Autodesk Fusion 360 part; units mm, degrees
note: some values were not read from the file. Set by a fixed rule: which face or edge a step refers to.
(part 2 of 3)
sketch "Sketch8" plane through (0, 0, 5) normal (0, 0, 1) x (-1, 0, 0)
  line L0 (-17, 136) -> (-35, 136)
  line L1 (-35, 136) -> (-35, 130)
  line L2 (-35, 130) -> (-17, 130)
  line L3 (-17, 130) -> (-17, 128)
  line L4 (-17, 128) -> (-35, 128)
  line L5 (-35, 128) -> (-35, 122)
  line L6 (-35, 122) -> (-17, 122)
  line L7 (-17, 122) -> (-17, 120)
  line L8 (-17, 120) -> (-35, 120)
  line L9 (-35, 120) -> (-35, 114)
  line L10 (-35, 114) -> (-17, 114)
  line L11 (-17, 114) -> (-17, 112)
  line L12 (-17, 112) -> (-35, 112)
  line L13 (-35, 112) -> (-35, 106)
  line L14 (-35, 106) -> (-17, 106)
  line L15 (-17, 106) -> (-17, 104)
  line L16 (-17, 104) -> (-35, 104)
  line L17 (-35, 104) -> (-35, 98)
  line L18 (-35, 98) -> (-17, 98)
  line L19 (-17, 98) -> (-17, 96)
  line L20 (-17, 96) -> (-35, 96)
  line L21 (-35, 96) -> (-35, 90)
  line L22 (-35, 90) -> (-17, 90)
  line L23 (-17, 90) -> (-17, 88)
  line L24 (-17, 88) -> (-35, 88)
  line L25 (-35, 88) -> (-35, 82)
  line L26 (-35, 82) -> (-17, 82)
  line L27 (-17, 82) -> (-17, 80)
  line L28 (-17, 80) -> (-35, 80)
  line L29 (-35, 80) -> (-35, 74)
  line L30 (-35, 74) -> (-17, 74)
  line L31 (-17, 74) -> (-17, 72)
  line L32 (-17, 72) -> (-35, 72)
  line L33 (-35, 72) -> (-35, 66)
  line L34 (-35, 66) -> (-17, 66)
  line L35 (-17, 66) -> (-17, 64)
  line L36 (-17, 64) -> (-35, 64)
  line L37 (-35, 64) -> (-35, 58)
  line L38 (-35, 58) -> (-17, 58)
  line L39 (-17, 58) -> (-17, 56)
  line L40 (-17, 56) -> (-35, 56)
  line L41 (-35, 56) -> (-35, 50)
  line L42 (-35, 50) -> (-17, 50)
  line L43 (-17, 50) -> (-17, 48)
  line L44 (-17, 48) -> (-35, 48)
  line L45 (-35, 48) -> (-35, 42)
  line L46 (-35, 42) -> (-17, 42)
  line L47 (-17, 42) -> (-17, 40)
  line L48 (-17, 40) -> (-35, 40)
  line L49 (-35, 40) -> (-35, 34)
  line L50 (-35, 34) -> (-17, 34)
  line L51 (-17, 34) -> (-17, 32)
  line L52 (-17, 32) -> (-35, 32)
  line L53 (-35, 32) -> (-35, 26)
  line L54 (-35, 26) -> (-17, 26)
  line L55 (-17, 26) -> (-17, 24)
  line L56 (-17, 24) -> (-35, 24)
  line L57 (-35, 24) -> (-35, 18)
  line L58 (-35, 18) -> (-17, 18)
  line L59 (-17, 18) -> (-17, 16)
  line L60 (-17, 16) -> (-35, 16)
  line L61 (-35, 16) -> (-35, 10)
  line L62 (-35, 10) -> (-17, 10)
  line L63 (-17, 10) -> (-17, 8)
  line L64 (-17, 8) -> (-35, 8)
  line L65 (-35, 8) -> (-35, 2)
  line L66 (-35, 2) -> (-17, 2)
  line L67 (-17, 2) -> (-17, 0)
  line L68 (-17, 0) -> (-35, 0)
  line L69 (-35, 0) -> (-35, -6)
  line L70 (-35, -6) -> (-17, -6)
  line L71 (-17, -6) -> (-17, -8)
  line L72 (-17, -8) -> (-35, -8)
  line L73 (-35, -8) -> (-35, -14)
  line L74 (-35, -14) -> (-17, -14)
  line L75 (-17, -14) -> (-17, -16)
  line L76 (-17, -16) -> (-35, -16)
  line L77 (-35, -16) -> (-35, -22)
  line L78 (-35, -22) -> (-17, -22)
  line L79 (-17, -22) -> (-17, -24)
  line L80 (-17, -24) -> (-35, -24)
  line L81 (-35, -24) -> (-35, -25)
  line L82 (-35, -25) -> (25, -25)
  line L83 (25, -25) -> (25, -24)
  line L84 (25, -24) -> (7, -24)
  line L85 (7, -24) -> (7, -22)
  line L86 (7, -22) -> (25, -22)
  line L87 (25, -22) -> (25, -16)
  line L88 (25, -16) -> (7, -16)
  line L89 (7, -16) -> (7, -14)
  line L90 (7, -14) -> (25, -14)
  line L91 (25, -14) -> (25, -8)
  line L92 (25, -8) -> (7, -8)
  line L93 (7, -8) -> (7, -6)
  line L94 (7, -6) -> (25, -6)
  line L95 (25, -6) -> (25, 0)
  line L96 (25, 0) -> (7, 0)
  line L97 (7, 0) -> (7, 2)
  line L98 (7, 2) -> (25, 2)
  line L99 (25, 2) -> (25, 8)
  line L100 (25, 8) -> (7, 8)
  line L101 (7, 8) -> (7, 10)
  line L102 (7, 10) -> (25, 10)
  line L103 (25, 10) -> (25, 16)
  line L104 (25, 16) -> (7, 16)
  line L105 (7, 16) -> (7, 18)
  line L106 (7, 18) -> (25, 18)
  line L107 (25, 18) -> (25, 24)
  line L108 (25, 24) -> (7, 24)
  line L109 (7, 24) -> (7, 26)
  line L110 (7, 26) -> (25, 26)
  line L111 (25, 26) -> (25, 32)
  line L112 (25, 32) -> (7, 32)
  line L113 (7, 32) -> (7, 34)
  line L114 (7, 34) -> (25, 34)
  line L115 (25, 34) -> (25, 40)
  line L116 (25, 40) -> (7, 40)
  line L117 (7, 40) -> (7, 42)
  line L118 (7, 42) -> (25, 42)
  line L119 (25, 42) -> (25, 48)
  line L120 (25, 48) -> (7, 48)
  line L121 (7, 48) -> (7, 50)
  line L122 (7, 50) -> (25, 50)
  line L123 (25, 50) -> (25, 56)
  line L124 (25, 56) -> (7, 56)
  line L125 (7, 56) -> (7, 58)
  line L126 (7, 58) -> (25, 58)
  line L127 (25, 58) -> (25, 64)
  line L128 (25, 64) -> (7, 64)
  line L129 (7, 64) -> (7, 66)
  line L130 (7, 66) -> (25, 66)
  line L131 (25, 66) -> (25, 72)
  line L132 (25, 72) -> (7, 72)
  line L133 (7, 72) -> (7, 74)
  line L134 (7, 74) -> (25, 74)
  line L135 (25, 74) -> (25, 80)
  line L136 (25, 80) -> (7, 80)
  line L137 (7, 80) -> (7, 82)
  line L138 (7, 82) -> (25, 82)
  line L139 (25, 82) -> (25, 88)
  line L140 (25, 88) -> (7, 88)
  line L141 (7, 88) -> (7, 90)
  line L142 (7, 90) -> (25, 90)
  line L143 (25, 90) -> (25, 96)
  line L144 (25, 96) -> (7, 96)
  line L145 (7, 96) -> (7, 98)
  line L146 (7, 98) -> (25, 98)
  line L147 (25, 98) -> (25, 104)
  line L148 (25, 104) -> (7, 104)
  line L149 (7, 104) -> (7, 106)
  line L150 (7, 106) -> (25, 106)
  line L151 (25, 106) -> (25, 112)
  line L152 (25, 112) -> (7, 112)
  line L153 (7, 112) -> (7, 114)
  line L154 (7, 114) -> (25, 114)
  line L155 (25, 114) -> (25, 120)
  line L156 (25, 120) -> (7, 120)
  line L157 (7, 120) -> (7, 122)
  line L158 (7, 122) -> (25, 122)
  line L159 (25, 122) -> (25, 128)
  line L160 (25, 128) -> (7, 128)
  line L161 (7, 128) -> (7, 130)
  line L162 (7, 130) -> (25, 130)
  line L163 (25, 130) -> (25, 136)
  line L164 (25, 136) -> (7, 136)
  line L165 (7, 136) -> (7, 138)
  line L166 (7, 138) -> (25, 138)
  line L167 (25, 138) -> (25, 150)
  line L168 (25, 150) -> (-35, 150)
  line L169 (-35, 150) -> (-35, 138)
  line L170 (-35, 138) -> (-17, 138)
  line L171 (-17, 138) -> (-17, 136)
  line L172 (23, 78) -> (23, 76)
  line L173 (23, 76) -> (-33, 76)
  line L174 (-33, 76) -> (-33, 78)
  line L175 (-33, 78) -> (23, 78)
  line L176 (-33, 94) -> (23, 94)
  line L177 (23, 94) -> (23, 92)
  line L178 (23, 92) -> (-33, 92)
  line L179 (-33, 92) -> (-33, 94)
  line L180 (23, 54) -> (23, 52)
  line L181 (23, 52) -> (-33, 52)
  line L182 (-33, 52) -> (-33, 54)
  line L183 (-33, 54) -> (23, 54)
  line L184 (4, 66) -> (4, 64)
  line L185 (4, 64) -> (-14, 64)
  line L186 (-14, 64) -> (-14, 66)
  line L187 (-14, 66) -> (4, 66)
  line L188 (4, 106) -> (4, 104)
  line L189 (4, 104) -> (-14, 104)
  line L190 (-14, 104) -> (-14, 106)
  line L191 (-14, 106) -> (4, 106)
  line L192 (23, 102) -> (23, 100)
  line L193 (23, 100) -> (-32.9874, 100)
  line L194 (-32.9874, 100) -> (-32.9874, 102)
  line L195 (-32.9874, 102) -> (23, 102)
  line L196 (4, 50) -> (4, 48)
  line L197 (4, 48) -> (-14, 48)
  line L198 (-14, 48) -> (-14, 50)
  line L199 (-14, 50) -> (4, 50)
  line L200 (4, 90) -> (4, 88)
  line L201 (4, 88) -> (-14, 88)
  line L202 (-14, 88) -> (-14, 90)
  line L203 (-14, 90) -> (4, 90)
  line L204 (4, 74) -> (4, 72)
  line L205 (4, 72) -> (-14, 72)
  line L206 (-14, 72) -> (-14, 74)
  line L207 (-14, 74) -> (4, 74)
  line L208 (23, 62) -> (23, 60)
  line L209 (23, 60) -> (-33, 60)
  line L210 (-33, 60) -> (-33, 62)
  line L211 (-33, 62) -> (23, 62)
  line L212 (-33, 116) -> (-33, 118)
  line L213 (-33, 118) -> (23, 118)
  line L214 (23, 118) -> (23, 116)
  line L215 (23, 116) -> (-33, 116)
  line L216 (4, 82) -> (4, 80)
  line L217 (4, 80) -> (-14, 80)
  line L218 (-14, 80) -> (-14, 82)
  line L219 (-14, 82) -> (4, 82)
  line L220 (4, 42) -> (4, 40)
  line L221 (4, 40) -> (-14, 40)
  line L222 (-14, 40) -> (-14, 42)
  line L223 (-14, 42) -> (4, 42)
  line L224 (23, 70) -> (23, 68)
  line L225 (23, 68) -> (-33, 68)
  line L226 (-33, 68) -> (-33, 70)
  line L227 (-33, 70) -> (23, 70)
  line L228 (23, 110) -> (23, 108)
  line L229 (23, 108) -> (-33, 108)
  line L230 (-33, 108) -> (-33, 110)
  line L231 (-33, 110) -> (23, 110)
  line L232 (4, 114) -> (4, 112)
  line L233 (4, 112) -> (-14, 112)
  line L234 (-14, 112) -> (-14, 114)
  line L235 (-14, 114) -> (4, 114)
  line L236 (4, 98) -> (4, 96)
  line L237 (4, 96) -> (-14, 96)
  line L238 (-14, 96) -> (-14, 98)
  line L239 (-14, 98) -> (4, 98)
  line L240 (23, 46.2715) -> (23, 44)
  line L241 (23, 44) -> (-33, 44)
  line L242 (-33, 44) -> (-33, 46.2715)
  line L243 (-33, 46.2715) -> (23, 46.2715)
  line L244 (23, 86) -> (23, 84)
  line L245 (23, 84) -> (-33, 84)
  line L246 (-33, 84) -> (-33, 86)
  line L247 (-33, 86) -> (23, 86)
  line L248 (4, 58) -> (4, 56)
  line L249 (4, 56) -> (-14, 56)
  line L250 (-14, 56) -> (-14, 58)
  line L251 (-14, 58) -> (4, 58)
  line L252 (23, -18) -> (23, -20)
  line L253 (23, -20) -> (-33, -20)
  line L254 (-33, -20) -> (-33, -18)
  line L255 (-33, -18) -> (23, -18)
  line L256 (4, -24) -> (-14, -24)
  line L257 (-14, -24) -> (-14, -22)
  line L258 (-14, -22) -> (4, -22)
  line L259 (4, -22) -> (4, -24)
  line L260 (23, 22) -> (23, 20)
  line L261 (23, 20) -> (-33, 20)
  line L262 (-33, 20) -> (-33, 22)
  line L263 (-33, 22) -> (23, 22)
  line L264 (23, 6) -> (23, 4)
  line L265 (23, 4) -> (-33, 4)
  line L266 (-33, 4) -> (-33, 6)
  line L267 (-33, 6) -> (23, 6)
  line L268 (23, -10) -> (23, -12)
  line L269 (23, -12) -> (-33, -12)
  line L270 (-33, -12) -> (-33, -10)
  line L271 (-33, -10) -> (23, -10)
  line L272 (4, -14) -> (4, -16)
  line L273 (4, -16) -> (-14, -16)
  line L274 (-14, -16) -> (-14, -14)
  line L275 (-14, -14) -> (4, -14)
  line L276 (4, -6) -> (4, -8)
  line L277 (4, -8) -> (-14, -8)
  line L278 (-14, -8) -> (-14, -6)
  line L279 (-14, -6) -> (4, -6)
  line L280 (4, 10) -> (4, 8)
  line L281 (4, 8) -> (-14, 8)
  line L282 (-14, 8) -> (-14, 10)
  line L283 (-14, 10) -> (4, 10)
  line L284 (4, 26) -> (4, 24)
  line L285 (4, 24) -> (-14, 24)
  line L286 (-14, 24) -> (-14, 26)
  line L287 (-14, 26) -> (4, 26)
  line L288 (4, 34) -> (4, 32)
  line L289 (4, 32) -> (-14, 32)
  line L290 (-14, 32) -> (-14, 34)
  line L291 (-14, 34) -> (4, 34)
  line L292 (4, 18) -> (4, 16)
  line L293 (4, 16) -> (-14, 16)
  line L294 (-14, 16) -> (-14, 18)
  line L295 (-14, 18) -> (4, 18)
  line L296 (4, 2) -> (4, 0)
  line L297 (4, 0) -> (-14, 0)
  line L298 (-14, 0) -> (-14, 2)
  line L299 (-14, 2) -> (4, 2)
  line L300 (23, 38) -> (23, 36)
  line L301 (23, 36) -> (-33, 36)
  line L302 (-33, 36) -> (-33, 38)
  line L303 (-33, 38) -> (23, 38)
  line L304 (23, -2) -> (23, -4)
  line L305 (23, -4) -> (-33, -4)
  line L306 (-33, -4) -> (-33, -2)
  line L307 (-33, -2) -> (23, -2)
  line L308 (23, 14) -> (23, 12)
  line L309 (23, 12) -> (-33, 12)
  line L310 (-33, 12) -> (-33, 14)
  line L311 (-33, 14) -> (23, 14)
  line L312 (23, 30) -> (23, 28)
  line L313 (23, 28) -> (-33, 28)
  line L314 (-33, 28) -> (-33, 30)
  line L315 (-33, 30) -> (23, 30)
  line L316 (4, 122) -> (4, 120)
  line L317 (4, 120) -> (-14, 120)
  line L318 (-14, 120) -> (-14, 122)
  line L319 (-14, 122) -> (4, 122)
  line L320 (4, 138) -> (4, 136)
  line L321 (4, 136) -> (-14, 136)
  line L322 (-14, 136) -> (-14, 138)
  line L323 (-14, 138) -> (4, 138)
  line L324 (4, 130) -> (4, 128)
  line L325 (4, 128) -> (-14, 128)
  line L326 (-14, 128) -> (-14, 130)
  line L327 (-14, 130) -> (4, 130)
  line L328 (23, 126) -> (23, 124)
  line L329 (23, 124) -> (-33, 124)
  line L330 (-33, 124) -> (-33, 126)
  line L331 (-33, 126) -> (23, 126)
  line L332 (23, 142) -> (23, 140)
  line L333 (23, 140) -> (-33, 140)
  line L334 (-33, 140) -> (-33, 142)
  line L335 (-33, 142) -> (23, 142)
  line L336 (23, 134) -> (23, 132)
  line L337 (23, 132) -> (-33, 132)
  line L338 (-33, 132) -> (-33, 134)
  line L339 (-33, 134) -> (23, 134)
  line L340 (25, 144) -> (25, 146)
  line L341 (25, 146) -> (7, 146)
  line L342 (7, 146) -> (7, 144)
  line L343 (7, 144) -> (25, 144)
  line L344 (4, 144) -> (4, 146)
  line L345 (4, 146) -> (-14, 146)
  line L346 (-14, 146) -> (-14, 144)
  line L347 (-14, 144) -> (4, 144)
  line L348 (-17, 144) -> (-17, 146)
  line L349 (-17, 146) -> (-35, 146)
  line L350 (-35, 146) -> (-35, 144)
  line L351 (-35, 144) -> (-17, 144)
  dimension "d102" = 18
  constraint perpendicular L340 L341
  constraint parallel L340 L342
  constraint parallel L341 L343
  constraint coincident L167 L340.end
  constraint midpoint L167 L340.start
  constraint perpendicular L344 L345
  constraint parallel L344 L346
  constraint parallel L345 L347
  constraint perpendicular L341 L344
  constraint perpendicular L348 L349
  constraint parallel L348 L350
  constraint parallel L349 L351
  constraint perpendicular L168 L348
  measures "d102" distance of L340.start L342.end
extrude "Extrude8" cut sketch "Sketch8" against normal blind 10 contours L169 L348 L349 L350 L351 | L167 L340 L341 L342 L343 | L344 L345 L346 L347
extrude "Extrude9" cut 1 faces at (15, -150, 1.6667) along direction (0, 1, 0) blind 3
extrude "Extrude10" add 1 faces at (15, -147, 1.6667) along direction (0, -1, 0) blind 20
extrude "Extrude11" add 1 faces at (-5, 25, 1.6667) along direction (0, 1, 0) blind 20
sketch "Sketch10" plane through (0, 0, 5) normal (0, 0, 1) x (-1, 0, 0)
  line L0 (4, 146) -> (4, 144)
  line L1 (4, 144) -> (-14, 144)
  line L2 (-14, 144) -> (-14, 146)
  line L3 (-14, 146) -> (4, 146)
  line L4 (23, 78) -> (23, 76)
  line L5 (23, 76) -> (-33, 76)
  line L6 (-33, 76) -> (-33, 78)
  line L7 (-33, 78) -> (23, 78)
  line L8 (-33, 94) -> (23, 94)
  line L9 (23, 94) -> (23, 92)
  line L10 (23, 92) -> (-33, 92)
  line L11 (-33, 92) -> (-33, 94)
  line L12 (23, 54) -> (23, 52)
  line L13 (23, 52) -> (-33, 52)
  line L14 (-33, 52) -> (-33, 54)
  line L15 (-33, 54) -> (23, 54)
  line L16 (4, 66) -> (4, 64)
  line L17 (4, 64) -> (-14, 64)
  line L18 (-14, 64) -> (-14, 66)
  line L19 (-14, 66) -> (4, 66)
  line L20 (4, 106) -> (4, 104)
  line L21 (4, 104) -> (-14, 104)
  line L22 (-14, 104) -> (-14, 106)
  line L23 (-14, 106) -> (4, 106)
  line L24 (23, 102) -> (23, 100)
  line L25 (23, 100) -> (-32.9874, 100)
  line L26 (-32.9874, 100) -> (-32.9874, 102)
  line L27 (-32.9874, 102) -> (23, 102)
  line L28 (4, 50) -> (4, 48)
  line L29 (4, 48) -> (-14, 48)
  line L30 (-14, 48) -> (-14, 50)
  line L31 (-14, 50) -> (4, 50)
  line L32 (4, 90) -> (4, 88)
  line L33 (4, 88) -> (-14, 88)
  line L34 (-14, 88) -> (-14, 90)
  line L35 (-14, 90) -> (4, 90)
  line L36 (4, 74) -> (4, 72)
  line L37 (4, 72) -> (-14, 72)
  line L38 (-14, 72) -> (-14, 74)
  line L39 (-14, 74) -> (4, 74)
  line L40 (23, 62) -> (23, 60)
  line L41 (23, 60) -> (-33, 60)
  line L42 (-33, 60) -> (-33, 62)
  line L43 (-33, 62) -> (23, 62)
  line L44 (-33, 116) -> (-33, 118)
  line L45 (-33, 118) -> (23, 118)
  line L46 (23, 118) -> (23, 116)
  line L47 (23, 116) -> (-33, 116)
  line L48 (4, 82) -> (4, 80)
  line L49 (4, 80) -> (-14, 80)
  line L50 (-14, 80) -> (-14, 82)
  line L51 (-14, 82) -> (4, 82)
  line L52 (4, 42) -> (4, 40)
  line L53 (4, 40) -> (-14, 40)
  line L54 (-14, 40) -> (-14, 42)
  line L55 (-14, 42) -> (4, 42)
  line L56 (23, 70) -> (23, 68)
  line L57 (23, 68) -> (-33, 68)
  line L58 (-33, 68) -> (-33, 70)
  line L59 (-33, 70) -> (23, 70)
  line L60 (23, 110) -> (23, 108)
  line L61 (23, 108) -> (-33, 108)
  line L62 (-33, 108) -> (-33, 110)
  line L63 (-33, 110) -> (23, 110)
  line L64 (4, 114) -> (4, 112)
  line L65 (4, 112) -> (-14, 112)
  line L66 (-14, 112) -> (-14, 114)
  line L67 (-14, 114) -> (4, 114)
  line L68 (4, 98) -> (4, 96)
  line L69 (4, 96) -> (-14, 96)
  line L70 (-14, 96) -> (-14, 98)
  line L71 (-14, 98) -> (4, 98)
  line L72 (23, 46.2715) -> (23, 44)
  line L73 (23, 44) -> (-33, 44)
  line L74 (-33, 44) -> (-33, 46.2715)
  line L75 (-33, 46.2715) -> (23, 46.2715)
  line L76 (23, 86) -> (23, 84)
  line L77 (23, 84) -> (-33, 84)
  line L78 (-33, 84) -> (-33, 86)
  line L79 (-33, 86) -> (23, 86)
  line L80 (4, 58) -> (4, 56)
  line L81 (4, 56) -> (-14, 56)
  line L82 (-14, 56) -> (-14, 58)
  line L83 (-14, 58) -> (4, 58)
  line L84 (23, -18) -> (23, -20)
  line L85 (23, -20) -> (-33, -20)
  line L86 (-33, -20) -> (-33, -18)
  line L87 (-33, -18) -> (23, -18)
  line L88 (4, -24) -> (-14, -24)
  line L89 (-14, -24) -> (-14, -22)
  line L90 (-14, -22) -> (4, -22)
  line L91 (4, -22) -> (4, -24)
  line L92 (23, 22) -> (23, 20)
  line L93 (23, 20) -> (-33, 20)
  line L94 (-33, 20) -> (-33, 22)
  line L95 (-33, 22) -> (23, 22)
  line L96 (23, 6) -> (23, 4)
  line L97 (23, 4) -> (-33, 4)
  line L98 (-33, 4) -> (-33, 6)
  line L99 (-33, 6) -> (23, 6)
  line L100 (23, -10) -> (23, -12)
  line L101 (23, -12) -> (-33, -12)
  line L102 (-33, -12) -> (-33, -10)
  line L103 (-33, -10) -> (23, -10)
  line L104 (4, -14) -> (4, -16)
  line L105 (4, -16) -> (-14, -16)
  line L106 (-14, -16) -> (-14, -14)
  line L107 (-14, -14) -> (4, -14)
  line L108 (4, -6) -> (4, -8)
  line L109 (4, -8) -> (-14, -8)
  line L110 (-14, -8) -> (-14, -6)
  line L111 (-14, -6) -> (4, -6)
  line L112 (4, 10) -> (4, 8)
  line L113 (4, 8) -> (-14, 8)
  line L114 (-14, 8) -> (-14, 10)
  line L115 (-14, 10) -> (4, 10)
  line L116 (4, 26) -> (4, 24)
  line L117 (4, 24) -> (-14, 24)
  line L118 (-14, 24) -> (-14, 26)
  line L119 (-14, 26) -> (4, 26)
  line L120 (4, 34) -> (4, 32)
  line L121 (4, 32) -> (-14, 32)
  line L122 (-14, 32) -> (-14, 34)
  line L123 (-14, 34) -> (4, 34)
  line L124 (4, 18) -> (4, 16)
  line L125 (4, 16) -> (-14, 16)
  line L126 (-14, 16) -> (-14, 18)
  line L127 (-14, 18) -> (4, 18)
  line L128 (4, 2) -> (4, 0)
  line L129 (4, 0) -> (-14, 0)
  line L130 (-14, 0) -> (-14, 2)
  line L131 (-14, 2) -> (4, 2)
  line L132 (23, 38) -> (23, 36)
  line L133 (23, 36) -> (-33, 36)
  line L134 (-33, 36) -> (-33, 38)
  line L135 (-33, 38) -> (23, 38)
  line L136 (23, -2) -> (23, -4)
  line L137 (23, -4) -> (-33, -4)
  line L138 (-33, -4) -> (-33, -2)
  line L139 (-33, -2) -> (23, -2)
  line L140 (23, 14) -> (23, 12)
  line L141 (23, 12) -> (-33, 12)
  line L142 (-33, 12) -> (-33, 14)
  line L143 (-33, 14) -> (23, 14)
  line L144 (23, 30) -> (23, 28)
  line L145 (23, 28) -> (-33, 28)
  line L146 (-33, 28) -> (-33, 30)
  line L147 (-33, 30) -> (23, 30)
  line L148 (4, 122) -> (4, 120)
  line L149 (4, 120) -> (-14, 120)
  line L150 (-14, 120) -> (-14, 122)
  line L151 (-14, 122) -> (4, 122)
  line L152 (4, 138) -> (4, 136)
  line L153 (4, 136) -> (-14, 136)
  line L154 (-14, 136) -> (-14, 138)
  line L155 (-14, 138) -> (4, 138)
  line L156 (4, 130) -> (4, 128)
  line L157 (4, 128) -> (-14, 128)
  line L158 (-14, 128) -> (-14, 130)
  line L159 (-14, 130) -> (4, 130)
  line L160 (23, 126) -> (23, 124)
  line L161 (23, 124) -> (-33, 124)
  line L162 (-33, 124) -> (-33, 126)
  line L163 (-33, 126) -> (23, 126)
  line L164 (23, 142) -> (23, 140)
  line L165 (23, 140) -> (-33, 140)
  line L166 (-33, 140) -> (-33, 142)
  line L167 (-33, 142) -> (23, 142)
  line L168 (23, 134) -> (23, 132)
  line L169 (23, 132) -> (-33, 132)
  line L170 (-33, 132) -> (-33, 134)
  line L171 (-33, 134) -> (23, 134)
  line L172 (-35, 167) -> (-35, 146)
  line L173 (-35, 146) -> (-17, 146)
  line L174 (-17, 146) -> (-17, 144)
  line L175 (-17, 144) -> (-35, 144)
  line L176 (-35, 144) -> (-35, 138)
  line L177 (-35, 138) -> (-17, 138)
  line L178 (-17, 138) -> (-17, 136)
  line L179 (-17, 136) -> (-35, 136)
  line L180 (-35, 136) -> (-35, 130)
  line L181 (-35, 130) -> (-17, 130)
  line L182 (-17, 130) -> (-17, 128)
  line L183 (-17, 128) -> (-35, 128)
  line L184 (-35, 128) -> (-35, 122)
  line L185 (-35, 122) -> (-17, 122)
  line L186 (-17, 122) -> (-17, 120)
  line L187 (-17, 120) -> (-35, 120)
  line L188 (-35, 120) -> (-35, 114)
  line L189 (-35, 114) -> (-17, 114)
  line L190 (-17, 114) -> (-17, 112)
  line L191 (-17, 112) -> (-35, 112)
  line L192 (-35, 112) -> (-35, 106)
  line L193 (-35, 106) -> (-17, 106)
  line L194 (-17, 106) -> (-17, 104)
  line L195 (-17, 104) -> (-35, 104)
  line L196 (-35, 104) -> (-35, 98)
  line L197 (-35, 98) -> (-17, 98)
  line L198 (-17, 98) -> (-17, 96)
  line L199 (-17, 96) -> (-35, 96)
  line L200 (-35, 96) -> (-35, 90)
  line L201 (-35, 90) -> (-17, 90)
  line L202 (-17, 90) -> (-17, 88)
  line L203 (-17, 88) -> (-35, 88)
  line L204 (-35, 88) -> (-35, 82)
  line L205 (-35, 82) -> (-17, 82)
  line L206 (-17, 82) -> (-17, 80)
  line L207 (-17, 80) -> (-35, 80)
  line L208 (-35, 80) -> (-35, 74)
  line L209 (-35, 74) -> (-17, 74)
  line L210 (-17, 74) -> (-17, 72)
  line L211 (-17, 72) -> (-35, 72)
  line L212 (-35, 72) -> (-35, 66)
  line L213 (-35, 66) -> (-17, 66)
  line L214 (-17, 66) -> (-17, 64)
  line L215 (-17, 64) -> (-35, 64)
  line L216 (-35, 64) -> (-35, 58)
  line L217 (-35, 58) -> (-17, 58)
  line L218 (-17, 58) -> (-17, 56)
  line L219 (-17, 56) -> (-35, 56)
  line L220 (-35, 56) -> (-35, 50)
  line L221 (-35, 50) -> (-17, 50)
  line L222 (-17, 50) -> (-17, 48)
  line L223 (-17, 48) -> (-35, 48)
  line L224 (-35, 48) -> (-35, 42)
  line L225 (-35, 42) -> (-17, 42)
  line L226 (-17, 42) -> (-17, 40)
  line L227 (-17, 40) -> (-35, 40)
  line L228 (-35, 40) -> (-35, 34)
  line L229 (-35, 34) -> (-17, 34)
  line L230 (-17, 34) -> (-17, 32)
  line L231 (-17, 32) -> (-35, 32)
  line L232 (-35, 32) -> (-35, 26)
  line L233 (-35, 26) -> (-17, 26)
  line L234 (-17, 26) -> (-17, 24)
  line L235 (-17, 24) -> (-35, 24)
  line L236 (-35, 24) -> (-35, 18)
  line L237 (-35, 18) -> (-17, 18)
  line L238 (-17, 18) -> (-17, 16)
  line L239 (-17, 16) -> (-35, 16)
  line L240 (-35, 16) -> (-35, 10)
  line L241 (-35, 10) -> (-17, 10)
  line L242 (-17, 10) -> (-17, 8)
  line L243 (-17, 8) -> (-35, 8)
  line L244 (-35, 8) -> (-35, 2)
  line L245 (-35, 2) -> (-17, 2)
  line L246 (-17, 2) -> (-17, 0)
  line L247 (-17, 0) -> (-35, 0)
  line L248 (-35, 0) -> (-35, -6)
  line L249 (-35, -6) -> (-17, -6)
  line L250 (-17, -6) -> (-17, -8)
  line L251 (-17, -8) -> (-35, -8)
  line L252 (-35, -8) -> (-35, -14)
  line L253 (-35, -14) -> (-17, -14)
  line L254 (-17, -14) -> (-17, -16)
  line L255 (-17, -16) -> (-35, -16)
  line L256 (-35, -16) -> (-35, -22)
  line L257 (-35, -22) -> (-17, -22)
  line L258 (-17, -22) -> (-17, -24)
  line L259 (-17, -24) -> (-35, -24)
  line L260 (-35, -24) -> (-35, -45)
  line L261 (-35, -45) -> (25, -45)
  line L262 (25, -45) -> (25, -24)
  line L263 (25, -24) -> (7, -24)
  line L264 (7, -24) -> (7, -22)
  line L265 (7, -22) -> (25, -22)
  line L266 (25, -22) -> (25, -16)
  line L267 (25, -16) -> (7, -16)
  line L268 (7, -16) -> (7, -14)
  line L269 (7, -14) -> (25, -14)
  line L270 (25, -14) -> (25, -8)
  line L271 (25, -8) -> (7, -8)
  line L272 (7, -8) -> (7, -6)
  line L273 (7, -6) -> (25, -6)
  line L274 (25, -6) -> (25, 0)
  line L275 (25, 0) -> (7, 0)
  line L276 (7, 0) -> (7, 2)
  line L277 (7, 2) -> (25, 2)
  line L278 (25, 2) -> (25, 8)
  line L279 (25, 8) -> (7, 8)
  line L280 (7, 8) -> (7, 10)
  line L281 (7, 10) -> (25, 10)
  line L282 (25, 10) -> (25, 16)
  line L283 (25, 16) -> (7, 16)
  line L284 (7, 16) -> (7, 18)
  line L285 (7, 18) -> (25, 18)
  line L286 (25, 18) -> (25, 24)
  line L287 (25, 24) -> (7, 24)
  line L288 (7, 24) -> (7, 26)
  line L289 (7, 26) -> (25, 26)
  line L290 (25, 26) -> (25, 32)
  line L291 (25, 32) -> (7, 32)
  line L292 (7, 32) -> (7, 34)
  line L293 (7, 34) -> (25, 34)
  line L294 (25, 34) -> (25, 40)
  line L295 (25, 40) -> (7, 40)
  line L296 (7, 40) -> (7, 42)
  line L297 (7, 42) -> (25, 42)
  line L298 (25, 42) -> (25, 48)
  line L299 (25, 48) -> (7, 48)
  line L300 (7, 48) -> (7, 50)
  line L301 (7, 50) -> (25, 50)
  line L302 (25, 50) -> (25, 56)
  line L303 (25, 56) -> (7, 56)
  line L304 (7, 56) -> (7, 58)
  line L305 (7, 58) -> (25, 58)
  line L306 (25, 58) -> (25, 64)
  line L307 (25, 64) -> (7, 64)
  line L308 (7, 64) -> (7, 66)
  line L309 (7, 66) -> (25, 66)
  line L310 (25, 66) -> (25, 72)
  line L311 (25, 72) -> (7, 72)
  line L312 (7, 72) -> (7, 74)
  line L313 (7, 74) -> (25, 74)
  line L314 (25, 74) -> (25, 80)
  line L315 (25, 80) -> (7, 80)
  line L316 (7, 80) -> (7, 82)
  line L317 (7, 82) -> (25, 82)
  line L318 (25, 82) -> (25, 88)
  line L319 (25, 88) -> (7, 88)
  line L320 (7, 88) -> (7, 90)
  line L321 (7, 90) -> (25, 90)
  line L322 (25, 90) -> (25, 96)
  line L323 (25, 96) -> (7, 96)
  line L324 (7, 96) -> (7, 98)
  line L325 (7, 98) -> (25, 98)
  line L326 (25, 98) -> (25, 104)
  line L327 (25, 104) -> (7, 104)
  line L328 (7, 104) -> (7, 106)
  line L329 (7, 106) -> (25, 106)
  line L330 (25, 106) -> (25, 112)
  line L331 (25, 112) -> (7, 112)
  line L332 (7, 112) -> (7, 114)
  line L333 (7, 114) -> (25, 114)
  line L334 (25, 114) -> (25, 120)
  line L335 (25, 120) -> (7, 120)
  line L336 (7, 120) -> (7, 122)
  line L337 (7, 122) -> (25, 122)
  line L338 (25, 122) -> (25, 128)
  line L339 (25, 128) -> (7, 128)
  line L340 (7, 128) -> (7, 130)
  line L341 (7, 130) -> (25, 130)
  line L342 (25, 130) -> (25, 136)
  line L343 (25, 136) -> (7, 136)
  line L344 (7, 136) -> (7, 138)
  line L345 (7, 138) -> (25, 138)
  line L346 (25, 138) -> (25, 144)
  line L347 (25, 144) -> (7, 144)
  line L348 (7, 144) -> (7, 146)
  line L349 (7, 146) -> (25, 146)
  line L350 (25, 146) -> (25, 167)
  line L351 (25, 167) -> (-35, 167)
  line L352 (23, -27) -> (23, -29)
  line L353 (23, -29) -> (-33, -29)
  line L354 (-33, -29) -> (-33, -27)
  line L355 (-33, -27) -> (23, -27)
  line L356 (25, -32) -> (25, -34)
  line L357 (25, -34) -> (7, -34)
  line L358 (7, -34) -> (7, -32)
  line L359 (7, -32) -> (25, -32)
  line L360 (4, -34) -> (4, -32)
  line L361 (4, -32) -> (-14, -32)
  line L362 (-14, -32) -> (-14, -34)
  line L363 (-14, -34) -> (4, -34)
  line L364 (-17, -34) -> (-17, -32)
  line L365 (-17, -32) -> (-35, -32)
  line L366 (-35, -32) -> (-35, -34)
  line L367 (-35, -34) -> (-17, -34)
  line L368 (23, -37) -> (23, -39)
  line L369 (23, -39) -> (-33, -39)
  line L370 (-33, -39) -> (-33, -37)
  line L371 (-33, -37) -> (23, -37)
  line L372 (25, -42) -> (25, -44)
  line L373 (25, -44) -> (7, -44)
  line L374 (7, -44) -> (7, -42)
  line L375 (7, -42) -> (25, -42)
  line L376 (4, -42) -> (4, -44)
  line L377 (4, -44) -> (-14, -44)
  line L378 (-14, -44) -> (-14, -42)
  line L379 (-14, -42) -> (4, -42)
  line L380 (-17, -42) -> (-17, -44)
  line L381 (-17, -44) -> (-35, -44)
  line L382 (-35, -44) -> (-35, -42)
  line L383 (-35, -42) -> (-17, -42)
  dimension "d111" = 56
  dimension "d112" = 18
  dimension "d113" = 18
  dimension "d114" = 18
  dimension "d115" = 56
  dimension "d116" = 18
  dimension "d117" = 18
  constraint perpendicular L352 L353
  constraint parallel L352 L354
  constraint parallel L353 L355
  constraint perpendicular L263 L352
  constraint perpendicular L356 L357
  constraint parallel L356 L358
  constraint parallel L357 L359
  constraint coincident L262 L356.end
  constraint coincident L262 L356.start
  constraint perpendicular L360 L361
  constraint parallel L360 L362
  constraint parallel L361 L363
  constraint perpendicular L357 L360
  constraint perpendicular L364 L365
  constraint parallel L364 L366
  constraint parallel L365 L367
  constraint perpendicular L105 L364
  constraint perpendicular L368 L369
  constraint parallel L368 L370
  constraint parallel L369 L371
  constraint perpendicular L357 L368
  constraint perpendicular L372 L373
  constraint parallel L372 L374
  constraint parallel L373 L375
  constraint perpendicular L265 L372
  constraint coincident L262 L372.start
  constraint perpendicular L376 L377
  constraint parallel L376 L378
  constraint parallel L377 L379
  constraint perpendicular L265 L376
  constraint perpendicular L380 L381
  constraint parallel L380 L382
  constraint parallel L381 L383
  constraint vertical L380
  measures "d111" distance of L352.start L354.end
  measures "d112" distance of L356.start L358.end
  measures "d113" distance of L360.start L362.end
  measures "d114" distance of L364.start L366.end
  measures "d115" distance of L368.start L370.end
  measures "d116" distance of L372.start L374.end
  measures "d117" distance of L376.start L378.end
extrude "Extrude12" cut sketch "Sketch10" against normal blind 10 contours L260 L364 L365 L366 L367 | L262 L356 L357 L358 L359 | L260 L380 L381 L382 L383 | L262 L372 L373 L374 L375 | L352 L353 L354 L355 | L360 L361 L362 L363 | L368 L369 L370 L371 | L376 L377 L378 L379
sketch "Sketch11" plane through (0, 0, 5) normal (0, 0, 1) x (-1, 0, 0)
  line L0 (7, -32) -> (25, -32)
  line L1 (25, -32) -> (25, -24)
  line L2 (25, -24) -> (7, -24)
  line L3 (7, -24) -> (7, -22)
  line L4 (7, -22) -> (25, -22)
  line L5 (25, -22) -> (25, -16)
  line L6 (25, -16) -> (7, -16)
  line L7 (7, -16) -> (7, -14)
  line L8 (7, -14) -> (25, -14)
  line L9 (25, -14) -> (25, -8)
  line L10 (25, -8) -> (7, -8)
  line L11 (7, -8) -> (7, -6)
  line L12 (7, -6) -> (25, -6)
  line L13 (25, -6) -> (25, 0)
  line L14 (25, 0) -> (7, 0)
  line L15 (7, 0) -> (7, 2)
  line L16 (7, 2) -> (25, 2)
  line L17 (25, 2) -> (25, 8)
  line L18 (25, 8) -> (7, 8)
  line L19 (7, 8) -> (7, 10)
  line L20 (7, 10) -> (25, 10)
  line L21 (25, 10) -> (25, 16)
  line L22 (25, 16) -> (7, 16)
  line L23 (7, 16) -> (7, 18)
  line L24 (7, 18) -> (25, 18)
  line L25 (25, 18) -> (25, 24)
  line L26 (25, 24) -> (7, 24)
  line L27 (7, 24) -> (7, 26)
  line L28 (7, 26) -> (25, 26)
  line L29 (25, 26) -> (25, 32)
  line L30 (25, 32) -> (7, 32)
  line L31 (7, 32) -> (7, 34)
  line L32 (7, 34) -> (25, 34)
  line L33 (25, 34) -> (25, 40)
  line L34 (25, 40) -> (7, 40)
  line L35 (7, 40) -> (7, 42)
  line L36 (7, 42) -> (25, 42)
  line L37 (25, 42) -> (25, 48)
  line L38 (25, 48) -> (7, 48)
  line L39 (7, 48) -> (7, 50)
  line L40 (7, 50) -> (25, 50)
  line L41 (25, 50) -> (25, 56)
  line L42 (25, 56) -> (7, 56)
  line L43 (7, 56) -> (7, 58)
  line L44 (7, 58) -> (25, 58)
  line L45 (25, 58) -> (25, 64)
  line L46 (25, 64) -> (7, 64)
  line L47 (7, 64) -> (7, 66)
  line L48 (7, 66) -> (25, 66)
  line L49 (25, 66) -> (25, 72)
  line L50 (25, 72) -> (7, 72)
  line L51 (7, 72) -> (7, 74)
  line L52 (7, 74) -> (25, 74)
  line L53 (25, 74) -> (25, 80)
  line L54 (25, 80) -> (7, 80)
  line L55 (7, 80) -> (7, 82)
  line L56 (7, 82) -> (25, 82)
  line L57 (25, 82) -> (25, 88)
  line L58 (25, 88) -> (7, 88)
  line L59 (7, 88) -> (7, 90)
  line L60 (7, 90) -> (25, 90)
  line L61 (25, 90) -> (25, 96)
  line L62 (25, 96) -> (7, 96)
  line L63 (7, 96) -> (7, 98)
  line L64 (7, 98) -> (25, 98)
  line L65 (25, 98) -> (25, 104)
  line L66 (25, 104) -> (7, 104)
  line L67 (7, 104) -> (7, 106)
  line L68 (7, 106) -> (25, 106)
  line L69 (25, 106) -> (25, 112)
  line L70 (25, 112) -> (7, 112)
  line L71 (7, 112) -> (7, 114)
  line L72 (7, 114) -> (25, 114)
  line L73 (25, 114) -> (25, 120)
  line L74 (25, 120) -> (7, 120)
  line L75 (7, 120) -> (7, 122)
  line L76 (7, 122) -> (25, 122)
  line L77 (25, 122) -> (25, 128)
  line L78 (25, 128) -> (7, 128)
  line L79 (7, 128) -> (7, 130)
  line L80 (7, 130) -> (25, 130)
  line L81 (25, 130) -> (25, 136)
  line L82 (25, 136) -> (7, 136)
  line L83 (7, 136) -> (7, 138)
  line L84 (7, 138) -> (25, 138)
  line L85 (25, 138) -> (25, 144)
  line L86 (25, 144) -> (7, 144)
  line L87 (7, 144) -> (7, 146)
  line L88 (7, 146) -> (25, 146)
  line L89 (25, 146) -> (25, 167)
  line L90 (25, 167) -> (-35, 167)
  line L91 (-35, 167) -> (-35, 146)
  line L92 (-35, 146) -> (-17, 146)
  line L93 (-17, 146) -> (-17, 144)
  line L94 (-17, 144) -> (-35, 144)
  line L95 (-35, 144) -> (-35, 138)
  line L96 (-35, 138) -> (-17, 138)
  line L97 (-17, 138) -> (-17, 136)
  line L98 (-17, 136) -> (-35, 136)
  line L99 (-35, 136) -> (-35, 130)
  line L100 (-35, 130) -> (-17, 130)
  line L101 (-17, 130) -> (-17, 128)
  line L102 (-17, 128) -> (-35, 128)
  line L103 (-35, 128) -> (-35, 122)
  line L104 (-35, 122) -> (-17, 122)
  line L105 (-17, 122) -> (-17, 120)
  line L106 (-17, 120) -> (-35, 120)
  line L107 (-35, 120) -> (-35, 114)
  line L108 (-35, 114) -> (-17, 114)
  line L109 (-17, 114) -> (-17, 112)
  line L110 (-17, 112) -> (-35, 112)
  line L111 (-35, 112) -> (-35, 106)
  line L112 (-35, 106) -> (-17, 106)
  line L113 (-17, 106) -> (-17, 104)
  line L114 (-17, 104) -> (-35, 104)
  line L115 (-35, 104) -> (-35, 98)
  line L116 (-35, 98) -> (-17, 98)
  line L117 (-17, 98) -> (-17, 96)
  line L118 (-17, 96) -> (-35, 96)
  line L119 (-35, 96) -> (-35, 90)
  line L120 (-35, 90) -> (-17, 90)
  line L121 (-17, 90) -> (-17, 88)
  line L122 (-17, 88) -> (-35, 88)
  line L123 (-35, 88) -> (-35, 82)
  line L124 (-35, 82) -> (-17, 82)
  line L125 (-17, 82) -> (-17, 80)
  line L126 (-17, 80) -> (-35, 80)
  line L127 (-35, 80) -> (-35, 74)
  line L128 (-35, 74) -> (-17, 74)
  line L129 (-17, 74) -> (-17, 72)
  line L130 (-17, 72) -> (-35, 72)
  line L131 (-35, 72) -> (-35, 66)
  line L132 (-35, 66) -> (-17, 66)
  line L133 (-17, 66) -> (-17, 64)
  line L134 (-17, 64) -> (-35, 64)
  line L135 (-35, 64) -> (-35, 58)
  line L136 (-35, 58) -> (-17, 58)
  line L137 (-17, 58) -> (-17, 56)
  line L138 (-17, 56) -> (-35, 56)
  line L139 (-35, 56) -> (-35, 50)
  line L140 (-35, 50) -> (-17, 50)
  line L141 (-17, 50) -> (-17, 48)
  line L142 (-17, 48) -> (-35, 48)
  line L143 (-35, 48) -> (-35, 42)
  line L144 (-35, 42) -> (-17, 42)
  line L145 (-17, 42) -> (-17, 40)
  line L146 (-17, 40) -> (-35, 40)
  line L147 (-35, 40) -> (-35, 34)
  line L148 (-35, 34) -> (-17, 34)
  line L149 (-17, 34) -> (-17, 32)
  line L150 (-17, 32) -> (-35, 32)
  line L151 (-35, 32) -> (-35, 26)
  line L152 (-35, 26) -> (-17, 26)
  line L153 (-17, 26) -> (-17, 24)
  line L154 (-17, 24) -> (-35, 24)
  line L155 (-35, 24) -> (-35, 18)
  line L156 (-35, 18) -> (-17, 18)
  line L157 (-17, 18) -> (-17, 16)
  line L158 (-17, 16) -> (-35, 16)
  line L159 (-35, 16) -> (-35, 10)
  line L160 (-35, 10) -> (-17, 10)
  line L161 (-17, 10) -> (-17, 8)
  line L162 (-17, 8) -> (-35, 8)
  line L163 (-35, 8) -> (-35, 2)
  line L164 (-35, 2) -> (-17, 2)
  line L165 (-17, 2) -> (-17, 0)
  line L166 (-17, 0) -> (-35, 0)
  line L167 (-35, 0) -> (-35, -6)
  line L168 (-35, -6) -> (-17, -6)
  line L169 (-17, -6) -> (-17, -8)
  line L170 (-17, -8) -> (-35, -8)
  line L171 (-35, -8) -> (-35, -14)
  line L172 (-35, -14) -> (-17, -14)
  line L173 (-17, -14) -> (-17, -16)
  line L174 (-17, -16) -> (-35, -16)
  line L175 (-35, -16) -> (-35, -22)
  line L176 (-35, -22) -> (-17, -22)
  line L177 (-17, -22) -> (-17, -24)
  line L178 (-17, -24) -> (-35, -24)
  line L179 (-35, -24) -> (-35, -32)
  line L180 (-35, -32) -> (-17, -32)
  line L181 (-17, -32) -> (-17, -34)
  line L182 (-17, -34) -> (-35, -34)
  line L183 (-35, -34) -> (-35, -42)
  line L184 (-35, -42) -> (-17, -42)
  line L185 (-17, -42) -> (-17, -44)
  line L186 (-17, -44) -> (-35, -44)
  line L187 (-35, -44) -> (-35, -45)
  line L188 (-35, -45) -> (25, -45)
  line L189 (25, -45) -> (25, -44)
  line L190 (25, -44) -> (7, -44)
  line L191 (7, -44) -> (7, -42)
  line L192 (7, -42) -> (25, -42)
  line L193 (25, -42) -> (25, -34)
  line L194 (25, -34) -> (7, -34)
  line L195 (7, -34) -> (7, -32)
  line L196 (23, 134) -> (23, 132)
  line L197 (23, 132) -> (-33, 132)
  line L198 (-33, 132) -> (-33, 134)
  line L199 (-33, 134) -> (23, 134)
  line L200 (23, 142) -> (23, 140)
  line L201 (23, 140) -> (-33, 140)
  line L202 (-33, 140) -> (-33, 142)
  line L203 (-33, 142) -> (23, 142)
  line L204 (23, 126) -> (23, 124)
  line L205 (23, 124) -> (-33, 124)
  line L206 (-33, 124) -> (-33, 126)
  line L207 (-33, 126) -> (23, 126)
  line L208 (4, 130) -> (4, 128)
  line L209 (4, 128) -> (-14, 128)
  line L210 (-14, 128) -> (-14, 130)
  line L211 (-14, 130) -> (4, 130)
  line L212 (4, 138) -> (4, 136)
  line L213 (4, 136) -> (-14, 136)
  line L214 (-14, 136) -> (-14, 138)
  line L215 (-14, 138) -> (4, 138)
  line L216 (4, 122) -> (4, 120)
  line L217 (4, 120) -> (-14, 120)
  line L218 (-14, 120) -> (-14, 122)
  line L219 (-14, 122) -> (4, 122)
  line L220 (23, 30) -> (23, 28)
  line L221 (23, 28) -> (-33, 28)
  line L222 (-33, 28) -> (-33, 30)
  line L223 (-33, 30) -> (23, 30)
  line L224 (23, 14) -> (23, 12)
  line L225 (23, 12) -> (-33, 12)
  line L226 (-33, 12) -> (-33, 14)
  line L227 (-33, 14) -> (23, 14)
  line L228 (23, -2) -> (23, -4)
  line L229 (23, -4) -> (-33, -4)
  line L230 (-33, -4) -> (-33, -2)
  line L231 (-33, -2) -> (23, -2)
  line L232 (23, 38) -> (23, 36)
  line L233 (23, 36) -> (-33, 36)
  line L234 (-33, 36) -> (-33, 38)
  line L235 (-33, 38) -> (23, 38)
  line L236 (4, 2) -> (4, 0)
  line L237 (4, 0) -> (-14, 0)
  line L238 (-14, 0) -> (-14, 2)
  line L239 (-14, 2) -> (4, 2)
  line L240 (4, 18) -> (4, 16)
  line L241 (4, 16) -> (-14, 16)
  line L242 (-14, 16) -> (-14, 18)
  line L243 (-14, 18) -> (4, 18)
  line L244 (4, 34) -> (4, 32)
  line L245 (4, 32) -> (-14, 32)
  line L246 (-14, 32) -> (-14, 34)
  line L247 (-14, 34) -> (4, 34)
  line L248 (4, 26) -> (4, 24)
  line L249 (4, 24) -> (-14, 24)
  line L250 (-14, 24) -> (-14, 26)
  line L251 (-14, 26) -> (4, 26)
  line L252 (4, 10) -> (4, 8)
  line L253 (4, 8) -> (-14, 8)
  line L254 (-14, 8) -> (-14, 10)
  line L255 (-14, 10) -> (4, 10)
  line L256 (4, -6) -> (4, -8)
  line L257 (4, -8) -> (-14, -8)
  line L258 (-14, -8) -> (-14, -6)
  line L259 (-14, -6) -> (4, -6)
  line L260 (4, -14) -> (4, -16)
  line L261 (4, -16) -> (-14, -16)
  line L262 (-14, -16) -> (-14, -14)
  line L263 (-14, -14) -> (4, -14)
  line L264 (23, -10) -> (23, -12)
  line L265 (23, -12) -> (-33, -12)
  line L266 (-33, -12) -> (-33, -10)
  line L267 (-33, -10) -> (23, -10)
  line L268 (23, 6) -> (23, 4)
  line L269 (23, 4) -> (-33, 4)
  line L270 (-33, 4) -> (-33, 6)
  line L271 (-33, 6) -> (23, 6)
  line L272 (23, 22) -> (23, 20)
  line L273 (23, 20) -> (-33, 20)
  line L274 (-33, 20) -> (-33, 22)
  line L275 (-33, 22) -> (23, 22)
  line L276 (4, -24) -> (-14, -24)
  line L277 (-14, -24) -> (-14, -22)
  line L278 (-14, -22) -> (4, -22)
  line L279 (4, -22) -> (4, -24)
  line L280 (23, -18) -> (23, -20)
  line L281 (23, -20) -> (-33, -20)
  line L282 (-33, -20) -> (-33, -18)
  line L283 (-33, -18) -> (23, -18)
  line L284 (4, 58) -> (4, 56)
  line L285 (4, 56) -> (-14, 56)
  line L286 (-14, 56) -> (-14, 58)
  line L287 (-14, 58) -> (4, 58)
  line L288 (23, 86) -> (23, 84)
  line L289 (23, 84) -> (-33, 84)
  line L290 (-33, 84) -> (-33, 86)
  line L291 (-33, 86) -> (23, 86)
  line L292 (23, 46.2715) -> (23, 44)
  line L293 (23, 44) -> (-33, 44)
  line L294 (-33, 44) -> (-33, 46.2715)
  line L295 (-33, 46.2715) -> (23, 46.2715)
  line L296 (4, 98) -> (4, 96)
  line L297 (4, 96) -> (-14, 96)
  line L298 (-14, 96) -> (-14, 98)
  line L299 (-14, 98) -> (4, 98)
  line L300 (4, 114) -> (4, 112)
  line L301 (4, 112) -> (-14, 112)
  line L302 (-14, 112) -> (-14, 114)
  line L303 (-14, 114) -> (4, 114)
  line L304 (23, 110) -> (23, 108)
  line L305 (23, 108) -> (-33, 108)
  line L306 (-33, 108) -> (-33, 110)
  line L307 (-33, 110) -> (23, 110)
  line L308 (23, 70) -> (23, 68)
  line L309 (23, 68) -> (-33, 68)
  line L310 (-33, 68) -> (-33, 70)
  line L311 (-33, 70) -> (23, 70)
  line L312 (4, 42) -> (4, 40)
  line L313 (4, 40) -> (-14, 40)
  line L314 (-14, 40) -> (-14, 42)
  line L315 (-14, 42) -> (4, 42)
  line L316 (4, 82) -> (4, 80)
  line L317 (4, 80) -> (-14, 80)
  line L318 (-14, 80) -> (-14, 82)
  line L319 (-14, 82) -> (4, 82)
  line L320 (-33, 116) -> (-33, 118)
  line L321 (-33, 118) -> (23, 118)
  line L322 (23, 118) -> (23, 116)
  line L323 (23, 116) -> (-33, 116)
  line L324 (23, 62) -> (23, 60)
  line L325 (23, 60) -> (-33, 60)
  line L326 (-33, 60) -> (-33, 62)
  line L327 (-33, 62) -> (23, 62)
  line L328 (4, 74) -> (4, 72)
  line L329 (4, 72) -> (-14, 72)
  line L330 (-14, 72) -> (-14, 74)
  line L331 (-14, 74) -> (4, 74)
  line L332 (4, 90) -> (4, 88)
  line L333 (4, 88) -> (-14, 88)
  line L334 (-14, 88) -> (-14, 90)
  line L335 (-14, 90) -> (4, 90)
  line L336 (4, 50) -> (4, 48)
  line L337 (4, 48) -> (-14, 48)
  line L338 (-14, 48) -> (-14, 50)
  line L339 (-14, 50) -> (4, 50)
  line L340 (23, 102) -> (23, 100)
  line L341 (23, 100) -> (-32.9874, 100)
  line L342 (-32.9874, 100) -> (-32.9874, 102)
  line L343 (-32.9874, 102) -> (23, 102)
  line L344 (4, 106) -> (4, 104)
  line L345 (4, 104) -> (-14, 104)
  line L346 (-14, 104) -> (-14, 106)
  line L347 (-14, 106) -> (4, 106)
  line L348 (4, 66) -> (4, 64)
  line L349 (4, 64) -> (-14, 64)
  line L350 (-14, 64) -> (-14, 66)
  line L351 (-14, 66) -> (4, 66)
  line L352 (23, 54) -> (23, 52)
  line L353 (23, 52) -> (-33, 52)
  line L354 (-33, 52) -> (-33, 54)
  line L355 (-33, 54) -> (23, 54)
  line L356 (-33, 94) -> (23, 94)
  line L357 (23, 94) -> (23, 92)
  line L358 (23, 92) -> (-33, 92)
  line L359 (-33, 92) -> (-33, 94)
  line L360 (23, 78) -> (23, 76)
  line L361 (23, 76) -> (-33, 76)
  line L362 (-33, 76) -> (-33, 78)
  line L363 (-33, 78) -> (23, 78)
  line L364 (4, 146) -> (4, 144)
  line L365 (4, 144) -> (-14, 144)
  line L366 (-14, 144) -> (-14, 146)
  line L367 (-14, 146) -> (4, 146)
  line L368 (23, -39) -> (-33, -39)
  line L369 (-33, -39) -> (-33, -37)
  line L370 (-33, -37) -> (23, -37)
  line L371 (23, -37) -> (23, -39)
  line L372 (4, -32) -> (4, -34)
  line L373 (4, -34) -> (-14, -34)
  line L374 (-14, -34) -> (-14, -32)
  line L375 (-14, -32) -> (4, -32)
  line L376 (23, -29) -> (-33, -29)
  line L377 (-33, -29) -> (-33, -27)
  line L378 (-33, -27) -> (23, -27)
  line L379 (23, -27) -> (23, -29)
  line L380 (4, -44) -> (-14, -44)
  line L381 (-14, -44) -> (-14, -42)
  line L382 (-14, -42) -> (4, -42)
  line L383 (4, -42) -> (4, -44)
  line L384 (23, 149) -> (23, 151)
  line L385 (23, 151) -> (-33, 151)
  line L386 (-33, 151) -> (-33, 149)
  line L387 (-33, 149) -> (23, 149)
  line L388 (25, 154) -> (25, 156)
  line L389 (25, 156) -> (7, 156)
  line L390 (7, 156) -> (7, 154)
  line L391 (7, 154) -> (25, 154)
  line L392 (4, 154) -> (4, 156)
  line L393 (4, 156) -> (-14, 156)
  line L394 (-14, 156) -> (-14, 154)
  line L395 (-14, 154) -> (4, 154)
  line L396 (-17, 154) -> (-17, 156)
  line L397 (-17, 156) -> (-35, 156)
  line L398 (-35, 156) -> (-35, 154)
  line L399 (-35, 154) -> (-17, 154)
  line L400 (23, 159) -> (23, 161)
  line L401 (23, 161) -> (-33, 161)
  line L402 (-33, 161) -> (-33, 159)
  line L403 (-33, 159) -> (23, 159)
  line L404 (25, 164) -> (7, 164)
  line L405 (7, 164) -> (7, 166)
  line L406 (7, 166) -> (25, 166)
  line L407 (25, 166) -> (25, 164)
  line L408 (4, 164) -> (-14, 164)
  line L409 (-14, 164) -> (-14, 166)
  line L410 (-14, 166) -> (4, 166)
  line L411 (4, 166) -> (4, 164)
  line L412 (-17, 164) -> (-35, 164)
  line L413 (-35, 164) -> (-35, 166)
  line L414 (-35, 166) -> (-17, 166)
  line L415 (-17, 166) -> (-17, 164)
  dimension "d120" = 2
  dimension "d121" = 56
  dimension "d122" = 18
  dimension "d123" = 18
  dimension "d124" = 56
  constraint perpendicular L384 L385
  constraint parallel L384 L386
  constraint parallel L385 L387
  constraint vertical L384
  constraint perpendicular L388 L389
  constraint parallel L388 L390
  constraint parallel L389 L391
  constraint coincident L89 L388.end
  constraint coincident L89 L388.start
  constraint perpendicular L392 L393
  constraint parallel L392 L394
  constraint parallel L393 L395
  constraint perpendicular L391 L392
  constraint perpendicular L396 L397
  constraint parallel L396 L398
  constraint parallel L397 L399
  constraint perpendicular L393 L396
  constraint perpendicular L400 L401
  constraint parallel L400 L402
  constraint parallel L401 L403
  constraint perpendicular L389 L400
  constraint horizontal L404
  constraint vertical L405
  constraint horizontal L406
  constraint vertical L407
  constraint coincident L89 L404.start
  constraint horizontal L408
  constraint vertical L409
  constraint horizontal L410
  constraint vertical L411
  constraint horizontal L412
  constraint vertical L413
  constraint horizontal L414
  constraint vertical L415
  constraint coincident L91 L413.end
  measures "d120" distance of L384.start L384.end
  measures "d121" distance of L384.start L386.end
  measures "d122" distance of L388.start L390.end
  measures "d123" distance of L396.start L398.end
  measures "d124" distance of L400.start L402.end
extrude "Extrude13" cut sketch "Sketch11" against normal blind 10 contours L89 L388 L389 L390 L391 | L89 L404 L405 L406 L407 | L91 L412 L413 L414 L415 | L91 L396 L397 L398 L399 | L384 L385 L386 L387 | L392 L393 L394 L395 | L400 L401 L402 L403 | L408 L409 L410 L411
extrude "Extrude14" add 1 faces at (-25, 44.6667, 3.3333) along direction (-1, 0, 0) blind 5
extrude "Extrude15" add 1 faces at (35, 44.6667, 3.3333) along direction (1, 0, 0) blind 5
extrude "Extrude16" add 1 faces at (16.6667, 45, 3.3333) along direction (0, 1, 0) blind 25
extrude "Extrude17" add 1 faces at (24.6667, 44, 3.3333) along direction (0, -1, 0) blind 2
extrude "Extrude18" add 1 faces at (2, 44, 3.3333) along direction (0, -1, 0) blind 2
extrude "Extrude19" add 1 faces at (-14.6667, 44, 3.3333) along direction (0, -1, 0) blind 2